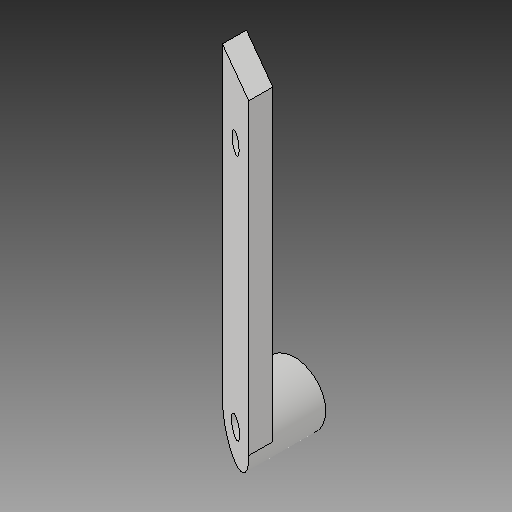
# Autodesk Inventor part: terminal_mount
Saved by Autodesk Inventor 2018 (Build 220112000, 112)
## iProperties
Created: 2017-06-03
Part Number: terminal_mount
Material: Generic
Document SubType Name: Modeling
Designer: AYUSH SHUKLA
Density: 1 g/cm^3
Appearance: Default
Author: AYUSH SHUKLA
Autodesk Inventor part; units mm, degrees
ref_plane "YZ Plane" through (0, 0, 0) normal (1, 0, 0) x (0, 1, 0)
ref_plane "XZ Plane" through (0, 0, 0) normal (0, 1, 0) x (-1, 0, 0)
ref_plane "XY Plane" through (0, 0, 0) normal (0, 0, 1) x (1, 0, 0)
sketch "Sketch1" plane through (0, 0, 0) normal (0, 1, 0) x (-1, 0, 0)
  line L0 (0, 14.6647) -> (-13, 22.1703)
  line L1 (0, 14.6647) -> (15.0111, 14.6647) construction
  line L2 (-13, 22.1703) -> (-13, 27.1703)
  line L3 (0, 19.6647) -> (0, 14.6647)
  line L4 (0, 0) -> (-28.4468, 0) construction
  line L5 (-13, -7.1591) -> (0, -14.6647)
  line L6 (0, -14.6647) -> (0, -19.6647)
  line L7 (-13, 27.1703) -> (0, 27.1703)
  line L8 (0, 27.1703) -> (0, 19.6647)
  line L9 (0, -19.6647) -> (-13, -19.6647)
  line L10 (-13, -19.6647) -> (-13, -7.1591)
  point P0 (0, -12.7)
  dimension "d1" = 150
  dimension "d2" = 5
  dimension "d5" = 25.4
  dimension "d6" = 0
  dimension "d7" = 0
  dimension "d8" = 14.6647
  dimension "d9" = 13
  dimension "d10" = 13
  dimension "d11" = 5
  constraints: 22 end point, 4 horizontal, 2 perpendicular, 1 equal length, 1 parallel, 1 point on line, 1 vertical
  measures "d1" angle of L1 L0
  measures "d2" distance of L0.end L2.end
  measures "d5" distance between parallel lines of L5 L0
  measures "d6" distance between parallel lines of L3 L6
  measures "d7" distance from line of L4.start L6
  measures "d8" distance from line of L4.start L1
  measures "d9" distance of L6.end L9.end
  measures "d10" distance of L2.end L7.end
  measures "d11" distance of L5.end L6.end
extrude "Extrusion1" add sketch "Sketch1" against normal blind 70.4
fillet "Fillet1" radius 6.5 4 edges at (0, -70.4, 20.9175) (13, -70.4, 24.6703) (13, -70.4, -13.4119) (0, -70.4, -17.1647)
sketch "Sketch2" plane through (0, 0, 27.1703) normal (0, 0, 1) x (1, 0, 0)
  arc A0 (0, -63.9) -> (13, -63.9) centre (6.5, -63.9) ccw projected
  line L0 (0, -63.9) -> (0, 0) projected
  line L1 (0, 0) -> (13, 0) projected
  line L2 (13, 0) -> (13, -63.9) projected
  circle A1 centre (6.5, -63.9) radius 6.5
  constraints: 1 centre point, 1 coincident, 1 concentric
extrude "Extrusion2" add sketch "Sketch2" against normal blind 16 contours A1 A0
sketch "Sketch3" plane through (13, 0, -19.6647) normal (0, 0, -1) x (-1, 0, 0)
  arc A0 (0, -63.9) -> (13, -63.9) centre (6.5, -63.9) ccw projected
  line L0 (0, -63.9) -> (0, 0) projected
  line L1 (0, 0) -> (13, 0) projected
  line L2 (13, 0) -> (13, -63.9) projected
  circle A1 centre (6.5, -63.9) radius 6.5
  constraints: 1 centre point, 1 coincident
extrude "Extrusion3" add sketch "Sketch3" against normal blind 16 contours A1 A0
sketch "Sketch4" plane through (0, 0, 0) normal (0, 1, 0) x (1, 0, 0)
  line L0 (0, -14.6647) -> (13, -22.1703) projected
  line L1 (13, -22.1703) -> (13, -27.1703) projected
  line L2 (13, -27.1703) -> (0, -27.1703) projected
  line L3 (0, -27.1703) -> (0, -14.6647) projected
  line L4 (13, 7.1591) -> (0, 14.6647) projected
  line L5 (0, 14.6647) -> (0, 19.6647) projected
  line L6 (0, 19.6647) -> (13, 19.6647) projected
  line L7 (13, 19.6647) -> (13, 7.1591) projected
  line L8 (13, -27.1703) -> (0, -19.6647)
  line L9 (13, -27.1703) -> (28.0111, -27.1703) construction
  line L10 (0, 19.6647) -> (13, 12.1591)
  point P0 (0, 0)
  dimension "d19" = 150
  constraints: 6 end point, 2 point on line, 1 equal length, 1 horizontal
  measures "d19" angle of L9 L8
extrude "Extrusion4" cut sketch "Sketch4" against normal through all contours L8 L2 L3 | L10 L6 L7
sketch "Sketch5" plane through (13, -63.9, 27.1703) normal (-0.5, 0, 0.8660254) x (0.8660254, 0, 0.5)
  ellipse E0 centre (-7.5056, 0) end of major axis (-15.0111, 0) minor radius 6.5 (-15.0111, 0) -> (0, 0) ccw projected
  line L0 (-15.0111, 0) -> (-15.0111, 63.9) projected
  line L1 (-15.0111, 63.9) -> (0, 63.9) projected
  line L2 (0, 63.9) -> (0, 0) projected
  circle A0 centre (-7.5056, 51.2) radius 2
  point P0 (-24.8435, 63.9)
  dimension "d22" = 4
  dimension "d23" = 12.7
  constraints: 1 centre point, 1 other
  measures "d22" diameter of A0
  measures "d23" distance from line of A0.centre L1
extrude "Extrusion5" cut sketch "Sketch5" against normal up to next contours A0
sketch "Sketch6" plane through (0, -63.9, -19.6647) normal (0.5, 0, -0.8660254) x (-0.8660254, 0, -0.5)
  ellipse E0 centre (-7.5056, 0) end of major axis (-15.0111, 0) minor radius 6.5 (-15.0111, 0) -> (0, 0) ccw projected
  line L0 (-15.0111, 0) -> (-15.0111, 63.9) projected
  line L1 (-15.0111, 63.9) -> (0, 63.9) projected
  line L2 (0, 63.9) -> (0, 0) projected
  circle A0 centre (-7.5056, 51.2) radius 2
  point P0 (-9.8323, 63.9)
  dimension "d26" = 4
  dimension "d27" = 12.7
  constraints: 1 centre point, 1 other
  measures "d26" diameter of A0
  measures "d27" distance from line of L1 A0.centre
extrude "Extrusion6" cut sketch "Sketch6" against normal up to next contours A0
sketch "Sketch7" plane through (6.5, -63.9, -3.6647) normal (0, 0, 1) x (1, 0, 0)
  circle A0 centre (0, 0) radius 6.5 projected
  circle A1 centre (0, 0) radius 2
  point P0 (-6.5, 63.9)
  dimension "d30" = 4
  constraints: 1 centre point, 1 coincident
  measures "d30" diameter of A1
extrude "Extrusion7" cut sketch "Sketch7" along normal through all both and the other way through all contours A1
sketch "Sketch9" plane through (0, 0, 0) normal (0, 1, 0) x (1, 0, 0)
  line L0 (-2.3389, 1.3365) -> (18.6443, 1.3365)
  line L1 (18.6443, 1.3365) -> (18.6443, 23.2553)
  line L2 (18.6443, 23.2553) -> (-2.3389, 23.2553)
  line L3 (-2.3389, 23.2553) -> (-2.3389, 1.3365)
  point P0 (0, 0)
  constraints: 8 end point, 2 parallel, 1 horizontal, 1 perpendicular
extrude "Extrusion8" cut sketch "Sketch9" against normal through all
body "Solid1"
